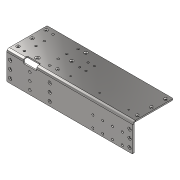
# Autodesk Inventor part: CCM_Mount_B
Saved by Autodesk Inventor 2020 (Build 240168000, 168)
## iProperties
Created: 2021-12-05
Part Number: CCM_Mount_B
Material: ステンレス鋼
Document SubType Name: Sheet Metal
Designer: ken113
Density: 8 g/cm^3
Sheet Metal Rule: Default_mm
Appearance: 半つや出し
Mass: 1103.55 g
Surface Area: 970.933 cm^2
Volume: 137.943 cm^3
Author: ken113
Autodesk Inventor part; units mm, degrees
ref_plane "YZ Plane" through (0, 0, 0) normal (1, 0, 0) x (0, 1, 0)
ref_plane "XZ Plane" through (0, 0, 0) normal (0, 1, 0) x (-1, 0, 0)
ref_plane "XY Plane" through (0, 0, 0) normal (0, 0, 1) x (1, 0, 0)
sketch "スケッチ1" plane through (0, 0, 0) normal (0, 0, 1) x (1, 0, 0)
  line L0 (150, -33.5) -> (-150, -33.5)
  line L1 (-150, -33.5) -> (-150, 33.5)
  line L2 (-150, 33.5) -> (150, 33.5)
  line L3 (150, 33.5) -> (150, -33.5)
  line L4 (150, -33.5) -> (-150, 33.5) construction
  line L5 (-150, -33.5) -> (150, 33.5) construction
  point P0 (0, 0)
  dimension "d1" = 67
  dimension "d2" = 300
  measures "d1" distance of L2.end L0.start
  measures "d2" distance of L0.start L0.end
extrude "プレート1" add sketch "スケッチ1" along normal blind 3
sketch "スケッチ2" plane through (150, 30.5, 3) normal (0, 1, 0) x (-1, 0, 0)
  line L0 (300, 0) -> (0, 0)
  line L1 (0, 0) -> (0, -96)
  line L2 (0, -96) -> (300, -96)
  line L3 (300, -96) -> (300, 0)
  constraints: 6 end point, 1 horizontal, 1 perpendicular, 1 vertical
edge flange "フランジ1" height 96 angle 90 thickness 3 bend radius 3 thickness toward (0, 1, 0) relief straight relief width 3 relief depth 1.5 edges at (0, 33.5, 0) wall of the first edge with corners at (-150, 30.5, 3) (150, 30.5, 3) (150, 30.5, -93) (-150, 30.5, -93)
bend "曲げ1"
corner "コーナー1"
fillet "フィレット1" radius 2 4 edges at (-150, 32, -93) (150, 32, -93) (150, -33.5, 1.5) (-150, -33.5, 1.5)
sketch "スケッチ3" plane through (-150, 30.5, -3) normal (0, -1, 0) x (1, 0, 0)
  line L0 (81.5, -55) -> (28.5, -55)
  line L1 (28.5, -55) -> (28.5, -35)
  line L2 (28.5, -35) -> (81.5, -35)
  line L3 (81.5, -35) -> (81.5, -55)
  line L4 (81.5, -55) -> (28.5, -35) construction
  line L5 (28.5, -55) -> (81.5, -35) construction
  line L6 (25, -79) -> (85, -79)
  line L7 (85, -79) -> (85, -11)
  line L8 (85, -11) -> (25, -11)
  line L9 (25, -11) -> (25, -79)
  line L10 (25, -79) -> (85, -11) construction
  line L11 (85, -79) -> (25, -11) construction
  line L12 (0, 0) -> (0, -88) projected
  line L13 (2, -90) -> (298, -90) projected
  point P0 (150, 3)
  point P1 (55, -45)
  dimension "d15" = 53
  dimension "d16" = 20
  dimension "d17" = 60
  dimension "d18" = 68
  dimension "d20" = 45
  dimension "d28" = 55
  constraints: 24 end point, 4 midpoint, 4 parallel, 2 horizontal, 2 perpendicular
  measures "d15" distance of L1.end L2.end
  measures "d16" distance of L0.end L1.end
  measures "d17" distance of L7.end L8.end
  measures "d18" distance of L6.end L7.end
  measures "d20" distance from line of L13 point (55, -45)
  measures "d28" distance from line of point (55, -45) L12
hole "穴1" at (-125, 30.5, -82) at (-65, 30.5, -82) at (-125, 30.5, -14) at (-65, 30.5, -14) at (-68.5, 30.5, -38) at (-68.5, 30.5, -58) at (-121.5, 30.5, -58) at (-121.5, 30.5, -38) direction (0, 1, 0) diameter 5.2 end through all
sketch "スケッチ4" plane through (-150, 33.5, -3) normal (0, 1, 0) x (1, 0, 0)
  circle A0 centre (28.5, 55) radius 2.6 projected
  circle A1 centre (81.5, 35) radius 2.6 projected
  circle A2 centre (25, 11) radius 2.6 projected
  circle A3 centre (25, 79) radius 2.6 projected
  circle A4 centre (85, 79) radius 2.6 projected
  circle A5 centre (85, 11) radius 2.6 projected
  circle A6 centre (81.5, 55) radius 2.6 projected
  circle A7 centre (28.5, 35) radius 2.6 projected
  arc A8 (300, 88) -> (298, 90) centre (298, 88) ccw projected
  line L0 (2, 90) -> (298, 90) projected
  arc A9 (2, 90) -> (0, 88) centre (2, 88) ccw projected
  line L1 (0, 0) -> (0, 88) projected
  line L2 (0, 0) -> (300, 0) projected
  line L3 (300, 88) -> (300, 0) projected
  line L4 (102, 13) -> (8, 13)
  line L5 (8, 13) -> (8, 80)
  line L6 (8, 80) -> (102, 80)
  line L7 (102, 80) -> (102, 13)
  line L8 (102, 80) -> (292, 80)
  line L9 (292, 80) -> (292, 13)
  line L10 (292, 13) -> (102, 13)
  line L11 (102, 13) -> (102, 80)
  point P0 (150, -3)
  point P1 (292, 46.5)
  point P2 (102, 46.5)
  point P3 (8, 46.5)
  dimension "d29" = 8
  dimension "d30" = 10
  dimension "d31" = 13
  dimension "d39" = 8
  dimension "d40" = 17
  constraints: 16 end point, 4 parallel, 3 midpoint, 2 horizontal, 2 perpendicular, 1 horizontal alignment
  measures "d29" distance between parallel lines of L9 L3
  measures "d30" distance between parallel lines of L6 L0
  measures "d31" distance between parallel lines of L2 L4
  measures "d39" distance between parallel lines of L1 L5
  measures "d40" distance from line of L7 A5.centre
hole "穴2" at (142, 33.5, -49.5) at (-48, 33.5, -49.5) at (-142, 33.5, -49.5) at (142, 33.5, -83) at (-48, 33.5, -83) at (-142, 33.5, -83) at (-142, 33.5, -16) at (-48, 33.5, -16) at (142, 33.5, -16) direction (0, -1, 0) diameter 4.3 end through all countersink diameter 8 countersink angle 90
sketch "スケッチ5" plane through (0, 0, 3) normal (0, 0, 1) x (1, 0, 0)
  arc A0 (-150, -31.5) -> (-148, -33.5) centre (-148, -31.5) ccw projected
  line L0 (148, -33.5) -> (-148, -33.5) projected
  arc A1 (148, -33.5) -> (150, -31.5) centre (148, -31.5) ccw projected
  line L1 (150, 27.5) -> (150, -31.5) projected
  line L2 (150, 27.5) -> (-150, 27.5) projected
  line L3 (-150, -31.5) -> (-150, 27.5) projected
  line L4 (142, 14.5) -> (-142, 14.5)
  line L5 (-142, 14.5) -> (-142, -23.5)
  line L6 (-142, -23.5) -> (142, -23.5)
  line L7 (142, -23.5) -> (142, 14.5)
  line L8 (-142, -23.5) -> (-48, -23.5)
  line L9 (-48, -23.5) -> (-48, 14.5)
  line L10 (-48, 14.5) -> (-142, 14.5)
  line L11 (-142, 14.5) -> (-142, -23.5)
  line L12 (-146, 33.5) -> (-138, 33.5) projected
  line L13 (-52, 33.5) -> (-44, 33.5) projected
  line L14 (138, 33.5) -> (146, 33.5) projected
  point P0 (0, 0)
  point P1 (-48, -4.5)
  point P2 (-142, -4.5)
  point P3 (142, -4.5)
  dimension "d41" = 8
  dimension "d42" = 8
  dimension "d43" = 94
  dimension "d44" = 13
  dimension "d45" = 10
  constraints: 16 end point, 4 parallel, 3 midpoint, 2 horizontal, 2 perpendicular, 1 point on line
  measures "d41" distance between parallel lines of L7 L1
  measures "d42" distance between parallel lines of L3 L5
  measures "d43" distance between parallel lines of L5 L9
  measures "d44" distance between parallel lines of L10 L2
  measures "d45" distance between parallel lines of L0 L6
hole "穴3" at (-48, -4.5, 3) at (-142, -4.5, 3) at (142, -4.5, 3) at (142, 14.5, 3) at (-48, 14.5, 3) at (-142, 14.5, 3) at (-142, -23.5, 3) at (-48, -23.5, 3) at (142, -23.5, 3) direction (0, 0, -1) diameter 4.3 end through all countersink diameter 8 countersink angle 90
sketch "スケッチ6" plane through (0, 0, 0) normal (0, 0, -1) x (-1, 0, 0)
  line L0 (-55, -27) -> (-125, -27)
  line L1 (-125, -27) -> (-125, 0)
  line L2 (-125, 0) -> (-55, 0)
  line L3 (-55, 0) -> (-55, -27)
  line L4 (-55, -27) -> (-125, 0) construction
  line L5 (-125, -27) -> (-55, 0) construction
  line L6 (-148, -33.5) -> (148, -33.5) projected
  line L7 (-150, 27.5) -> (-150, -31.5) projected
  line L8 (-101.6667, -27) -> (-78.3333, -27)
  line L9 (-78.3333, -27) -> (-78.3333, 0)
  line L10 (-78.3333, 0) -> (-101.6667, 0)
  line L11 (-101.6667, 0) -> (-101.6667, -27)
  line L12 (-101.6667, -27) -> (-78.3333, 0) construction
  line L13 (-78.3333, -27) -> (-101.6667, 0) construction
  point P0 (0, 0)
  point P1 (-90, -13.5)
  point P2 (-42.5, -33.5)
  dimension "d53" = 6.5
  dimension "d54" = 27
  dimension "d55" = 25
  dimension "d56" = 107.5
  dimension "d58" = 70
  dimension "d59" = 23.3333
  constraints: 24 end point, 4 midpoint, 4 parallel, 2 coincident, 2 horizontal, 2 perpendicular, 2 point on line
  measures "d53" distance between parallel lines of L6 L0
  measures "d54" distance of L0.end L1.end
  measures "d55" distance between parallel lines of L7 L1
  measures "d56" distance from line of point (-42.5, -33.5) L7
  measures "d58" distance of L0.start L0.end
  measures "d59" distance between parallel lines of L11 L1
hole "穴4" at (55, -27, 0) at (55, 0, 0) at (78.3333, -27, 0) at (78.3333, 0, 0) at (101.6667, 0, 0) at (101.6667, -27, 0) at (125, -27, 0) at (125, 0, 0) direction (0, 0, 1) diameter 5.2 end through all
sketch "スケッチ7" plane through (-150, 33.5, -3) normal (0, 1, 0) x (1, 0, 0)
  line L0 (139.5, 43) -> (124.5, 43)
  line L1 (124.5, 43) -> (124.5, 63)
  line L2 (124.5, 63) -> (139.5, 63)
  line L3 (139.5, 63) -> (139.5, 43)
  circle A0 centre (102, 13) radius 4 projected
  point P0 (150, -3)
  point P1 (132, 43)
  dimension "d67" = 15
  dimension "d68" = 20
  dimension "d69" = 30
  dimension "d70" = 30
  constraints: 8 end point, 2 parallel, 1 horizontal, 1 midpoint, 1 perpendicular
  measures "d67" distance of L0.start L0.end
  measures "d68" distance of L2.end L0.start
  measures "d69" horizontal distance of A0.centre point (132, 43)
  measures "d70" distance from line of L0 A0.centre
hole "穴5" at (-10.5, 33.5, -46) at (-10.5, 33.5, -66) at (-25.5, 33.5, -46) at (-25.5, 33.5, -66) direction (0, -1, 0) diameter 4.3434 depth 16.265 tip angle 118 thread size "12-24 UNC" class "2B" standard "ANSI Unified Screw Threads"
sketch "スケッチ8" plane through (-150, 33.5, -3) normal (0, 1, 0) x (1, 0, 0)
  circle A0 centre (124.5, 43) radius 2.1717 projected
  circle A1 centre (139.5, 43) radius 2.1717 projected
  circle A2 centre (139.5, 63) radius 2.1717 projected
  circle A3 centre (124.5, 63) radius 2.1717 projected
  circle A4 centre (102, 13) radius 4 projected
  circle A5 centre (8, 80) radius 4 projected
  circle A6 centre (292, 80) radius 4 projected
  circle A7 centre (102, 46.5) radius 4 projected
  circle A8 centre (292, 46.5) radius 4 projected
  circle A9 centre (8, 46.5) radius 4 projected
  circle A10 centre (102, 80) radius 4 projected
  circle A11 centre (8, 13) radius 4 projected
  circle A12 centre (292, 13) radius 4 projected
  circle A13 centre (28.5, 55) radius 2.6 projected
  circle A14 centre (81.5, 35) radius 2.6 projected
  circle A15 centre (25, 11) radius 2.6 projected
  circle A16 centre (25, 79) radius 2.6 projected
  circle A17 centre (85, 79) radius 2.6 projected
  circle A18 centre (85, 11) radius 2.6 projected
  circle A19 centre (81.5, 55) radius 2.6 projected
  circle A20 centre (28.5, 35) radius 2.6 projected
  arc A21 (300, 88) -> (298, 90) centre (298, 88) ccw projected
  line L0 (2, 90) -> (298, 90) projected
  arc A22 (2, 90) -> (0, 88) centre (2, 88) ccw projected
  line L1 (0, 0) -> (0, 88) projected
  line L2 (0, 0) -> (300, 0) projected
  line L3 (300, 88) -> (300, 0) projected
  line L4 (300, -6) -> (0, -6) projected
  line L5 (71, -19.2453) -> (39, -19.2453)
  line L6 (39, -19.2453) -> (39, 4)
  line L7 (39, 4) -> (71, 4)
  line L8 (71, 4) -> (71, -19.2453)
  circle A23 centre (85, 11) radius 2.6 projected
  circle A24 centre (25, 11) radius 2.6 projected
  line L9 (85, 11) -> (25, 11)
  point P0 (150, -3)
  point P1 (55, -19.2453)
  point P2 (55, 11)
  dimension "d78" = 32
  dimension "d79" = 10
  constraints: 10 end point, 2 horizontal, 2 midpoint, 2 parallel, 1 perpendicular, 1 vertical alignment
  measures "d78" distance of L6.end L7.end
  measures "d79" distance between parallel lines of L4 L7
extrude "押し出し1" cut sketch "スケッチ8" against normal blind 10 contours L8 L4 L6 L2 | L2 L6 L7 L8 | L8 L5 L6 L4
fillet "フィレット2" radius 2 4 edges at (-79, 32, -7) (-79, 23.5, 1.5) (-111, 23.5, 1.5) (-111, 32, -7)
sketch "スケッチ9" plane through (0, 0, 3) normal (0, 0, 1) x (1, 0, 0)
  line L0 (-109, 23.5) -> (-81, 23.5) projected
  line L1 (-95, 23.5) -> (-95, -33.5)
  line L2 (148, -33.5) -> (-148, -33.5) projected
  point P0 (0, 0)
  point P1 (-95, 13.5)
  point P2 (-95, -23.5)
  point P3 (-95, -5)
  dimension "d83" = 10
  dimension "d84" = 10
  dimension "d85" = 18.5
  constraints: 3 point on line, 2 end point, 2 midpoint, 1 vertical
  measures "d83" distance from line of point (-95, 13.5) L0
  measures "d84" distance from line of point (-95, -23.5) L2
  measures "d85" distance of point (-95, -5) point (-95, -23.5)
hole "穴6" at (-95, 13.5, 3) at (-95, -23.5, 3) at (-95, -5, 3) direction (0, 0, -1) diameter 6.3 depth 3 tip angle 118
sketch "スケッチ10" plane through (-148, 33.5, -93) normal (0, 1, 0) x (1, 0, 0)
  line L0 (268, -76) -> (130, -76)
  circle A0 centre (122.5, -47) radius 2.1717 projected
  circle A1 centre (137.5, -47) radius 2.1717 projected
  line L1 (137.5, -47) -> (122.5, -47)
  line L2 (298, -96) -> (69, -96) projected
  line L3 (298, -2) -> (298, -90) projected
  point P0 (148, -93)
  point P1 (130, -47)
  point P2 (199, -76)
  dimension "d94" = 20
  dimension "d95" = 30
  constraints: 4 end point, 2 coincident, 2 horizontal, 2 midpoint, 1 vertical alignment
  measures "d94" distance between parallel lines of L0 L2
  measures "d95" distance from line of L0.start L3
hole "穴7" at (51, 33.5, -17) at (-18, 33.5, -17) at (120, 33.5, -17) direction (0, -1, 0) diameter 3.242 depth 11.8 tip angle 118 thread size "M4x0.7" class "6H" standard "ISO Metric profile"
sketch "スケッチ11" plane through (-148, 33.5, -93) normal (0, 1, 0) x (1, 0, 0)
  circle A0 centre (130, -76) radius 1.621 projected
  circle A1 centre (199, -76) radius 1.621 projected
  circle A2 centre (268, -76) radius 1.621 projected
  line L0 (69, -88) -> (69, -90) projected
  line L1 (69, -90) -> (298, -90) projected
  line L2 (298, -2) -> (298, -90) projected
  arc A3 (298, -2) -> (296, 0) centre (296, -2) ccw projected
  line L3 (0, 0) -> (296, 0) projected
  arc A4 (0, 0) -> (-2, -2) centre (0, -2) ccw projected
  line L4 (-2, -90) -> (-2, -2) projected
  line L5 (-2, -90) -> (37, -90) projected
  line L6 (37, -90) -> (37, -88) projected
  arc A5 (39, -86) -> (37, -88) centre (39, -88) ccw projected
  line L7 (39, -86) -> (67, -86) projected
  arc A6 (69, -88) -> (67, -86) centre (67, -88) ccw projected
  circle A7 centre (122.5, -47) radius 2.1717 projected
  circle A8 centre (137.5, -47) radius 2.1717 projected
  circle A9 centre (137.5, -27) radius 2.1717 projected
  circle A10 centre (122.5, -27) radius 2.1717 projected
  circle A11 centre (100, -77) radius 4 projected
  circle A12 centre (6, -10) radius 4 projected
  circle A13 centre (290, -10) radius 4 projected
  circle A14 centre (100, -43.5) radius 4 projected
  circle A15 centre (290, -43.5) radius 4 projected
  circle A16 centre (6, -43.5) radius 4 projected
  circle A17 centre (100, -10) radius 4 projected
  circle A18 centre (6, -77) radius 4 projected
  circle A19 centre (290, -77) radius 4 projected
  circle A20 centre (26.5, -35) radius 2.6 projected
  circle A21 centre (79.5, -55) radius 2.6 projected
  circle A22 centre (23, -79) radius 2.6 projected
  circle A23 centre (23, -11) radius 2.6 projected
  circle A24 centre (83, -11) radius 2.6 projected
  circle A25 centre (83, -79) radius 2.6 projected
  circle A26 centre (79.5, -35) radius 2.6 projected
  circle A27 centre (26.5, -55) radius 2.6 projected
  line L8 (39, -93) -> (67, -93) projected
  point P0 (148, -93)
  point P1 (53, -78)
  point P2 (53, -86)
  dimension "d103" = 15
  constraints: 1 midpoint, 1 vertical alignment
  measures "d103" distance from line of point (53, -78) L8
hole "穴8" at (-95, 33.5, -15) direction (0, -1, 0) diameter 5.3 depth 3 tip angle 118 countersink diameter 10 countersink angle 90
equation "\"d26\" = Thickness"
equation "\"d37\" = Thickness"
equation "\"d51\" = Thickness"
equation "\"d59\" = 0.333333 * d58"
equation "\"d65\" = Thickness"
equation "\"d91\" = Thickness"
equation "\"d109\" = Thickness"
equation "\"d3\" = Thickness"
equation "\"d4\" = BendReliefWidth"
equation "\"d5\" = BendReliefDepth"
equation "\"d6\" = MinimumRemnant"
equation "\"d7\" = TransitionRadius"
equation "\"d10\" = BendRadius"
equation "\"d11\" = CornerReliefSize"
equation "\"d12\" = GapSize"
equation "\"d13\" = JacobiRadiusSize"
equation "\"BendRadius\" = Thickness"
equation "\"BendReliefWidth\" = Thickness"
equation "\"BendReliefDepth\" = 0.5 * Thickness"
equation "\"CornerReliefSize\" = 4 * Thickness"
equation "\"MinimumRemnant\" = 2 * Thickness"
equation "\"TransitionRadius\" = BendRadius"
equation "\"JacobiRadiusSize\" = BendRadius"
equation "\"GapSize\" = Thickness"
equation "\"Thickness\" = 3"
